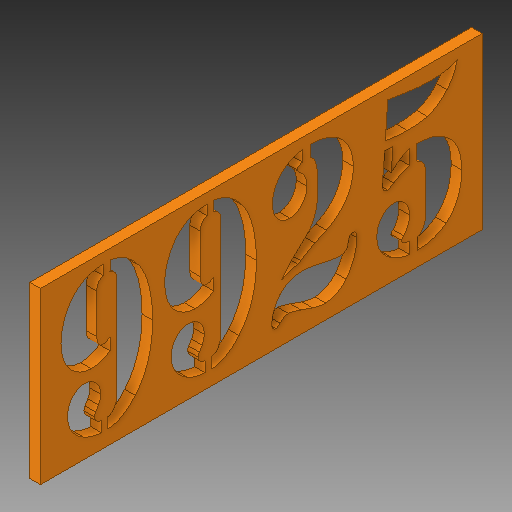
# Autodesk Inventor part: Numbers
Saved by Autodesk Inventor 2019 (Build 230136000, 136)
## iProperties
Created: 2017-10-20
Part Number: Numbers
Material: Generic
Document SubType Name: Modeling
Designer: User
Density: 1 g/cm^3
Appearance: Orange
Author: User
Autodesk Inventor part; units mm, degrees
ref_plane "YZ Plane" through (0, 0, 0) normal (1, 0, 0) x (0, 1, 0)
ref_plane "XZ Plane" through (0, 0, 0) normal (0, 1, 0) x (-1, 0, 0)
ref_plane "XY Plane" through (0, 0, 0) normal (0, 0, 1) x (1, 0, 0)
sketch "Sketch1" plane through (0, 0, 0) normal (1, 0, 0) x (0, 1, 0)
  line L0 (0, 0) -> (76.2, 0)
  line L1 (76.2, 0) -> (76.2, -215.9)
  line L2 (76.2, -215.9) -> (0, -215.9)
  line L3 (0, -215.9) -> (0, 0)
  dimension "d0" = 76.2
  dimension "d1" = 215.9
  constraints: 8 end point, 2 parallel, 1 horizontal, 1 perpendicular
  measures "d0" distance of L1.end L2.end
  measures "d1" distance of L0.end L1.end
extrude "Extrusion1" add sketch "Sketch1" along normal blind 4.7625
sketch "Sketch2" plane through (4.7625, 0, 0) normal (1, 0, 0) x (0, 0, -1)
  line L0 (15.9447, 71.619) -> (269.7922, 71.619) construction
  line L1 (269.7922, 71.619) -> (269.7922, 7.8945) construction
  line L2 (269.7922, 7.8945) -> (15.9447, 7.8945) construction
  line L3 (15.9447, 7.8945) -> (15.9447, 71.619) construction
  line L4 (0, 76.2) -> (0, 0) projected
  line L5 (0, 0) -> (215.9, 0) projected
  line L6 (215.9, 0) -> (215.9, 76.2) projected
  line L7 (215.9, 76.2) -> (0, 76.2) projected
  line L8 (39.1508, 6.5756) -> (39.1508, 11.261)
  spline S0 degree 2 poles (39.1508, 11.261) (40.4186, 11.7019) (41.7415, 12.7492) (42.1825, 13.7414) knots 0 0 0 1 2 2 2
  spline S1 degree 2 poles (42.1825, 13.7414) (43.1747, 15.6707) (43.1747, 17.9858) knots 0 0 0 1 1 1
  line L9 (43.1747, 17.9858) -> (43.1747, 60.9255)
  spline S2 degree 2 poles (43.1747, 60.9255) (43.1747, 63.0752) (42.9542, 64.8942) (42.5132, 65.5557) knots 0 0 0 1 2 2 2
  spline S3 degree 2 poles (42.5132, 65.5557) (41.9069, 66.4927) (40.0879, 67.0991) knots 0 0 0 1 1 1
  line L10 (40.0879, 67.0991) -> (40.0879, 71.619)
  spline S4 degree 2 poles (40.0879, 71.619) (43.8913, 71.1781) (50.5058, 66.8235) (53.0966, 63.1303) knots 0 0 0 1 2 2 2
  spline S5 degree 2 poles (53.0966, 63.1303) (56.018, 59.0513) (59.215, 46.208) (59.215, 38.7115) knots 0 0 0 1 2 2 2
  spline S6 degree 2 poles (59.215, 38.7115) (59.215, 22.7262) (51.4429, 13.4107) knots 0 0 0 1 1 1
  spline S7 degree 2 poles (51.4429, 13.4107) (48.6868, 10.1585) (42.2927, 6.5756) (39.1508, 6.5756) knots 0 0 0 1 2 2 2
  line L11 (40.0879, 41.7432) -> (40.0879, 36.3964)
  spline S8 degree 2 poles (40.0879, 36.3964) (35.7884, 33.6403) (31.7094, 33.6403) knots 0 0 0 1 1 1
  spline S9 degree 2 poles (31.7094, 33.6403) (29.2841, 33.6403) (24.3231, 35.9003) (22.449, 37.8295) knots 0 0 0 1 2 2 2
  spline S10 degree 2 poles (22.449, 37.8295) (20.4095, 40.0344) (18.0944, 46.4285) (18.0944, 50.0665) knots 0 0 0 1 2 2 2
  spline S11 degree 2 poles (18.0944, 50.0665) (18.0944, 55.2479) (22.1734, 64.9493) (25.5358, 67.7054) knots 0 0 0 1 2 2 2
  spline S12 degree 2 poles (25.5358, 67.7054) (30.4416, 71.619) (37.1113, 71.619) knots 0 0 0 1 1 1
  line L12 (37.1113, 71.619) -> (37.1113, 67.0991)
  spline S13 degree 2 poles (37.1113, 67.0991) (35.5679, 66.603) (34.1348, 64.5635) (34.1348, 62.5791) knots 0 0 0 1 2 2 2
  line L13 (34.1348, 62.5791) -> (34.1348, 44.8851)
  spline S14 degree 2 poles (34.1348, 44.8851) (34.1348, 42.7905) (35.6782, 40.4202) (36.946, 40.4754) knots 0 0 0 1 2 2 2
  spline S15 degree 2 poles (36.946, 40.4754) (38.1035, 40.5305) (40.0879, 41.7432) knots 0 0 0 1 1 1
  line L14 (36.1743, 11.261) -> (36.1743, 6.5756)
  spline S16 degree 2 poles (36.1743, 6.5756) (32.2606, 6.5756) (28.2368, 8.7805) knots 0 0 0 1 1 1
  spline S17 degree 2 poles (28.2368, 8.7805) (24.8192, 10.7097) (21.0158, 16.7731) (21.0158, 20.3009) knots 0 0 0 1 2 2 2
  spline S18 degree 2 poles (21.0158, 20.3009) (21.0158, 24.1594) (25.4256, 29.3959) (28.788, 29.3959) knots 0 0 0 1 2 2 2
  spline S19 degree 2 poles (28.788, 29.3959) (31.7094, 29.3959) (35.8435, 24.876) (35.8435, 21.6789) knots 0 0 0 1 2 2 2
  spline S20 degree 2 poles (35.8435, 21.6789) (35.8435, 19.4741) (34.9065, 17.9307) knots 0 0 0 1 1 1
  line L15 (34.9065, 17.9307) -> (33.6387, 15.836)
  spline S21 degree 2 poles (33.6387, 15.836) (33.1426, 14.9541) (33.1426, 14.1824) knots 0 0 0 1 1 1
  spline S22 degree 2 poles (33.1426, 14.1824) (33.1426, 12.8595) (34.3552, 11.8673) knots 0 0 0 1 1 1
  spline S23 degree 2 poles (34.3552, 11.8673) (34.9616, 11.3712) (36.1743, 11.261) knots 0 0 0 1 1 1
  line L16 (85.6734, 6.5756) -> (85.6734, 11.261)
  spline S24 degree 2 poles (85.6734, 11.261) (86.9412, 11.7019) (88.2641, 12.7492) (88.7051, 13.7414) knots 0 0 0 1 2 2 2
  spline S25 degree 2 poles (88.7051, 13.7414) (89.6973, 15.6707) (89.6973, 17.9858) knots 0 0 0 1 1 1
  line L17 (89.6973, 17.9858) -> (89.6973, 60.9255)
  spline S26 degree 2 poles (89.6973, 60.9255) (89.6973, 63.0752) (89.4768, 64.8942) (89.0358, 65.5557) knots 0 0 0 1 2 2 2
  spline S27 degree 2 poles (89.0358, 65.5557) (88.4295, 66.4927) (86.6104, 67.0991) knots 0 0 0 1 1 1
  line L18 (86.6104, 67.0991) -> (86.6104, 71.619)
  spline S28 degree 2 poles (86.6104, 71.619) (90.4138, 71.1781) (97.0284, 66.8235) (99.6191, 63.1303) knots 0 0 0 1 2 2 2
  spline S29 degree 2 poles (99.6191, 63.1303) (102.5406, 59.0513) (105.7376, 46.208) (105.7376, 38.7115) knots 0 0 0 1 2 2 2
  spline S30 degree 2 poles (105.7376, 38.7115) (105.7376, 22.7262) (97.9655, 13.4107) knots 0 0 0 1 1 1
  spline S31 degree 2 poles (97.9655, 13.4107) (95.2094, 10.1585) (88.8153, 6.5756) (85.6734, 6.5756) knots 0 0 0 1 2 2 2
  line L19 (86.6104, 41.7432) -> (86.6104, 36.3964)
  spline S32 degree 2 poles (86.6104, 36.3964) (82.311, 33.6403) (78.232, 33.6403) knots 0 0 0 1 1 1
  spline S33 degree 2 poles (78.232, 33.6403) (75.8066, 33.6403) (70.8457, 35.9003) (68.9716, 37.8295) knots 0 0 0 1 2 2 2
  spline S34 degree 2 poles (68.9716, 37.8295) (66.9321, 40.0344) (64.617, 46.4285) (64.617, 50.0665) knots 0 0 0 1 2 2 2
  spline S35 degree 2 poles (64.617, 50.0665) (64.617, 55.2479) (68.696, 64.9493) (72.0584, 67.7054) knots 0 0 0 1 2 2 2
  spline S36 degree 2 poles (72.0584, 67.7054) (76.9642, 71.619) (83.6339, 71.619) knots 0 0 0 1 1 1
  line L20 (83.6339, 71.619) -> (83.6339, 67.0991)
  spline S37 degree 2 poles (83.6339, 67.0991) (82.0905, 66.603) (80.6573, 64.5635) (80.6573, 62.5791) knots 0 0 0 1 2 2 2
  line L21 (80.6573, 62.5791) -> (80.6573, 44.8851)
  spline S38 degree 2 poles (80.6573, 44.8851) (80.6573, 42.7905) (82.2007, 40.4202) (83.4685, 40.4754) knots 0 0 0 1 2 2 2
  spline S39 degree 2 poles (83.4685, 40.4754) (84.6261, 40.5305) (86.6104, 41.7432) knots 0 0 0 1 1 1
  line L22 (82.6968, 11.261) -> (82.6968, 6.5756)
  spline S40 degree 2 poles (82.6968, 6.5756) (78.7832, 6.5756) (74.7593, 8.7805) knots 0 0 0 1 1 1
  spline S41 degree 2 poles (74.7593, 8.7805) (71.3418, 10.7097) (67.5384, 16.7731) (67.5384, 20.3009) knots 0 0 0 1 2 2 2
  spline S42 degree 2 poles (67.5384, 20.3009) (67.5384, 24.1594) (71.9481, 29.3959) (75.3105, 29.3959) knots 0 0 0 1 2 2 2
  spline S43 degree 2 poles (75.3105, 29.3959) (78.232, 29.3959) (82.3661, 24.876) (82.3661, 21.6789) knots 0 0 0 1 2 2 2
  spline S44 degree 2 poles (82.3661, 21.6789) (82.3661, 19.4741) (81.429, 17.9307) knots 0 0 0 1 1 1
  line L23 (81.429, 17.9307) -> (80.1612, 15.836)
  spline S45 degree 2 poles (80.1612, 15.836) (79.6651, 14.9541) (79.6651, 14.1824) knots 0 0 0 1 1 1
  spline S46 degree 2 poles (79.6651, 14.1824) (79.6651, 12.8595) (80.8778, 11.8673) knots 0 0 0 1 1 1
  spline S47 degree 2 poles (80.8778, 11.8673) (81.4841, 11.3712) (82.6968, 11.261) knots 0 0 0 1 1 1
  line L24 (129.8808, 66.5479) -> (129.8808, 71.619)
  line L25 (129.8808, 71.619) -> (130.9282, 71.619)
  spline S48 degree 2 poles (130.9282, 71.619) (135.0623, 71.619) (142.5588, 68.422) (145.0393, 65.5557) knots 0 0 0 1 2 2 2
  spline S49 degree 2 poles (145.0393, 65.5557) (149.2285, 60.7601) (149.2285, 53.4841) knots 0 0 0 1 1 1
  spline S50 degree 2 poles (149.2285, 53.4841) (149.2285, 47.2002) (142.9446, 37.4988) (137.1569, 34.7427) knots 0 0 0 1 2 2 2
  line L26 (137.1569, 34.7427) -> (131.9755, 32.3174)
  spline S51 degree 2 poles (131.9755, 32.3174) (129.7155, 31.2701) (125.6365, 28.6242) knots 0 0 0 1 1 1
  line L27 (125.6365, 28.6242) -> (124.4238, 27.7974)
  spline S52 degree 2 poles (124.4238, 27.7974) (122.8253, 27.7974) (119.9039, 26.8052) (117.1478, 25.4272) knots 0 0 0 1 2 2 2
  spline S53 degree 2 poles (117.1478, 25.4272) (118.5809, 27.6872) (121.4473, 30.9393) (124.3687, 33.5852) knots 0 0 0 1 2 2 2
  spline S54 degree 2 poles (124.3687, 33.5852) (128.0618, 36.9476) (130.6525, 39.9793) (131.5345, 42.0188) knots 0 0 0 1 2 2 2
  spline S55 degree 2 poles (131.5345, 42.0188) (132.4716, 44.0583) (133.2984, 49.5704) (133.2984, 53.8148) knots 0 0 0 1 2 2 2
  spline S56 degree 2 poles (133.2984, 53.8148) (133.2984, 61.2562) (132.196, 63.8469) knots 0 0 0 1 1 1
  spline S57 degree 2 poles (132.196, 63.8469) (131.755, 64.8942) (130.7628, 65.9966) (129.8808, 66.5479) knots 0 0 0 1 2 2 2
  spline S58 degree 2 poles (148.8427, 28.0179) (149.7246, 28.073) (150.8821, 26.3091) (150.8821, 24.876) knots 0 0 0 1 2 2 2
  spline S59 degree 2 poles (150.8821, 24.876) (150.8821, 21.6238) (148.0158, 13.6863) (145.9763, 11.261) knots 0 0 0 1 2 2 2
  spline S60 degree 2 poles (145.9763, 11.261) (144.2676, 9.1663) (139.0861, 6.5756) (136.8262, 6.5756) knots 0 0 0 1 2 2 2
  spline S61 degree 2 poles (136.8262, 6.5756) (134.0701, 6.5756) (130.9833, 7.6229) knots 0 0 0 1 1 1
  line L28 (130.9833, 7.6229) -> (125.7467, 9.442)
  spline S62 degree 2 poles (125.7467, 9.442) (121.337, 10.9302) (120.0692, 10.9302) knots 0 0 0 1 1 1
  spline S63 degree 2 poles (120.0692, 10.9302) (118.3053, 10.9302) (116.3761, 9.001) knots 0 0 0 1 1 1
  spline S64 degree 2 poles (116.3761, 9.001) (115.1634, 7.7883) (114.5019, 7.7883) knots 0 0 0 1 1 1
  spline S65 degree 2 poles (114.5019, 7.7883) (113.62, 7.7883) (112.6278, 9.1663) (112.6278, 10.4893) knots 0 0 0 1 2 2 2
  spline S66 degree 2 poles (112.6278, 10.4893) (112.6278, 12.9697) (114.6122, 18.2063) (116.321, 20.1355) knots 0 0 0 1 2 2 2
  spline S67 degree 2 poles (116.321, 20.1355) (119.9039, 24.2696) (126.0775, 24.2696) knots 0 0 0 1 1 1
  spline S68 degree 2 poles (126.0775, 24.2696) (128.9989, 24.2696) (133.9047, 23.2223) knots 0 0 0 1 1 1
  spline S69 degree 2 poles (133.9047, 23.2223) (141.0154, 21.6238) (143.2203, 21.6238) knots 0 0 0 1 1 1
  spline S70 degree 2 poles (143.2203, 21.6238) (145.0944, 21.6238) (146.0315, 22.7262) knots 0 0 0 1 1 1
  spline S71 degree 2 poles (146.0315, 22.7262) (146.3622, 23.1672) (146.6929, 24.2145) (146.9685, 25.6477) knots 0 0 0 1 2 2 2
  spline S72 degree 2 poles (146.9685, 25.6477) (147.4095, 27.9077) (148.8427, 28.0179) knots 0 0 0 1 1 1
  line L29 (126.4082, 71.5088) -> (126.4082, 66.5479)
  spline S73 degree 2 poles (126.4082, 66.5479) (125.3058, 66.2722) (123.9277, 65.2801) (123.9828, 64.7288) knots 0 0 0 1 2 2 2
  spline S74 degree 2 poles (123.9828, 64.7288) (124.038, 64.1225) (125.0302, 63.3508) knots 0 0 0 1 1 1
  spline S75 degree 2 poles (125.0302, 63.3508) (126.794, 61.9176) (128.3926, 58.5552) (128.3926, 56.185) knots 0 0 0 1 2 2 2
  spline S76 degree 2 poles (128.3926, 56.185) (128.3926, 52.6572) (123.8726, 47.5309) (120.7858, 47.5309) knots 0 0 0 1 2 2 2
  spline S77 degree 2 poles (120.7858, 47.5309) (117.4234, 47.5309) (112.9034, 52.988) (112.9034, 57.0118) knots 0 0 0 1 2 2 2
  spline S78 degree 2 poles (112.9034, 57.0118) (112.9034, 60.8152) (116.817, 67.4298) (120.1795, 69.359) knots 0 0 0 1 2 2 2
  spline S79 degree 2 poles (120.1795, 69.359) (122.3292, 70.5717) (126.4082, 71.5088) knots 0 0 0 1 1 1
  line L30 (177.7263, 41.2471) -> (177.7263, 47.9719)
  spline S80 degree 2 poles (177.7263, 47.9719) (181.8053, 47.9719) (187.3726, 46.4836) (189.9082, 44.7197) knots 0 0 0 1 2 2 2
  spline S81 degree 2 poles (189.9082, 44.7197) (197.8457, 39.2627) (197.8457, 27.7423) knots 0 0 0 1 1 1
  spline S82 degree 2 poles (197.8457, 27.7423) (197.8457, 22.175) (194.2077, 13.3556) (190.8453, 10.5995) knots 0 0 0 1 2 2 2
  spline S83 degree 2 poles (190.8453, 10.5995) (188.475, 8.7805) (182.2463, 6.5756) (179.1044, 6.5756) knots 0 0 0 1 2 2 2
  line L31 (179.1044, 6.5756) -> (177.8917, 6.5756)
  line L32 (177.8917, 6.5756) -> (177.8917, 11.8122)
  spline S84 degree 2 poles (177.8917, 11.8122) (179.1044, 12.2531) (180.5927, 13.7414) (181.0336, 15.0092) knots 0 0 0 1 2 2 2
  spline S85 degree 2 poles (181.0336, 15.0092) (181.3644, 15.7809) (181.8053, 19.0882) (181.8053, 20.6316) knots 0 0 0 1 2 2 2
  line L33 (181.8053, 20.6316) -> (181.8053, 32.5379)
  spline S86 degree 2 poles (181.8053, 32.5379) (181.8053, 36.6169) (180.1517, 40.1998) (177.7263, 41.2471) knots 0 0 0 1 2 2 2
  line L34 (163.5601, 56.2401) -> (164.6625, 71.619)
  spline S87 degree 2 poles (164.6625, 71.619) (165.9303, 71.4537) (166.2059, 71.3985) knots 0 0 0 1 1 1
  line L35 (166.2059, 71.3985) -> (174.1986, 70.1859)
  spline S88 degree 2 poles (174.1986, 70.1859) (178.3878, 69.4693) (184.2858, 69.4693) knots 0 0 0 1 1 1
  spline S89 degree 2 poles (184.2858, 69.4693) (188.2545, 69.4693) (193.1604, 70.4064) (195.8613, 71.619) knots 0 0 0 1 2 2 2
  spline S90 degree 2 poles (195.8613, 71.619) (195.0345, 68.422) (193.0501, 64.343) (191.2311, 62.2484) knots 0 0 0 1 2 2 2
  spline S91 degree 2 poles (191.2311, 62.2484) (189.357, 59.9884) (184.7268, 56.8465) (182.4117, 56.2401) knots 0 0 0 1 2 2 2
  spline S92 degree 2 poles (182.4117, 56.2401) (178.939, 55.3031) (173.4269, 55.3031) knots 0 0 0 1 1 1
  spline S93 degree 2 poles (173.4269, 55.3031) (168.4108, 55.3031) (163.5601, 56.2401) knots 0 0 0 1 1 1
  line L36 (174.419, 11.8122) -> (174.419, 6.6859)
  spline S94 degree 2 poles (174.419, 6.6859) (170.2849, 7.0166) (166.702, 9.2215) knots 0 0 0 1 1 1
  spline S95 degree 2 poles (166.702, 9.2215) (163.3396, 11.261) (159.7567, 17.159) (159.7567, 20.6867) knots 0 0 0 1 2 2 2
  spline S96 degree 2 poles (159.7567, 20.6867) (159.7567, 24.7106) (164.1664, 30.1125) (167.4737, 30.1125) knots 0 0 0 1 2 2 2
  spline S97 degree 2 poles (167.4737, 30.1125) (170.34, 30.1125) (174.4742, 25.2618) (174.4742, 21.9545) knots 0 0 0 1 2 2 2
  spline S98 degree 2 poles (174.4742, 21.9545) (174.4742, 20.0804) (172.8756, 16.2219) (171.7732, 15.2297) knots 0 0 0 1 2 2 2
  spline S99 degree 2 poles (171.7732, 15.2297) (170.8361, 14.4029) (170.8361, 13.9068) knots 0 0 0 1 1 1
  spline S100 degree 2 poles (170.8361, 13.9068) (170.8361, 13.1351) (172.7103, 12.0327) (174.419, 11.8122) knots 0 0 0 1 2 2 2
  line L37 (163.2845, 52.6572) -> (166.9225, 52.2163)
  line L38 (166.9225, 52.2163) -> (166.2611, 42.57)
  spline S101 degree 2 poles (166.2611, 42.57) (168.5762, 44.83) (172.2142, 47.1451) (174.419, 47.8065) knots 0 0 0 1 2 2 2
  line L39 (174.419, 47.8065) -> (174.419, 41.2471)
  spline S102 degree 2 poles (174.419, 41.2471) (170.1747, 40.0895) (167.3084, 37.9949) knots 0 0 0 1 1 1
  spline S103 degree 2 poles (167.3084, 37.9949) (165.3791, 36.6169) (164.5523, 36.6169) knots 0 0 0 1 1 1
  spline S104 degree 2 poles (164.5523, 36.6169) (163.4499, 36.6169) (162.2372, 37.9949) (162.2372, 39.1525) knots 0 0 0 1 2 2 2
  spline S105 degree 2 poles (162.2372, 39.1525) (162.2372, 39.7037) (162.2923, 40.4202) knots 0 0 0 1 1 1
  line L40 (162.2923, 40.4202) -> (163.2845, 52.6572)
  constraints: 2 other
extrude "Extrusion3" cut sketch "Sketch2" against normal blind 6.35 contours L8 S0 S1 L9 S2 S3 L10 S4 S5 S6 S7 | L11 S8 S9 S10 S11 S12 L12 S13 L13 S14 S15 | L14 S16 S17 S18 S19 S20 L15 S21 S22 S23 | L16 S24 S25 L17 S26 S27 L18 S28 S29 S30 S31 | L19 S32 S33 S34 S35 S36 L20 S37 L21 S38 S39 | L22 S40 S41 S42 S43 S44 L23 S45 S46 S47 | L24 L25 S48 S49 S50 L26 S51 L27 S52 S53 S54 S55 S56 S57 | S58 S59 S60 S61 L28 S62 S63 S64 S65 S66 S67 S68 S69 S70 S71 S72 | L29 S73 S74 S75 S76 S77 S78 S79 | L30 S80 S81 S82 S83 L31 L32 S84 S85 L33 S86 | L34 S87 L35 S88 S89 S90 S91 S92 S93 | L36 S94 S95 S96 S97 S98 S99 S100 | L37 L38 S101 L39 S102 S103 S104 S105 L40
thicken "Thicken1" operation add thickness 8.89 both sides no extend neighbours yes toward (0, 0, -1) faces at (1.5875, 25.4, 0)
thicken "Thicken2" operation add thickness 8.89 both sides no extend neighbours yes toward (0, 0, 1) faces at (1.5875, 50.8, -215.9)
body "Solid1"
